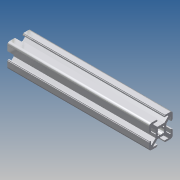
# Autodesk Inventor part: Motedius_20x20_B-Type_Slot-6_120
Saved by Autodesk Inventor 2015 SP1 (Build 190203100, 203)
## iProperties
Created: 2015-01-03
Part Number: Motedius_20x20_B-Type_Slot-6_120
Material: Aluminium 6061
Document SubType Name: Modeling
Designer: Marc
Mass: 190.994 g
Surface Area: 703.631 cm^2
Volume: 70.7386 cm^3
Density: 2.7 g/cm^3
Appearance: Aluminium - flach
Author: Marc
Autodesk Inventor part; units mm, degrees
ref_plane "YZ Plane" through (0, 0, 0) normal (1, 0, 0) x (0, 1, 0)
ref_plane "XZ Plane" through (0, 0, 0) normal (0, 1, 0) x (-1, 0, 0)
ref_plane "XY Plane" through (0, 0, 0) normal (0, 0, 1) x (1, 0, 0)
sketch "Skizze1" plane through (0, 0, 0) normal (1, 0, 0) x (0, 1, 0)
  line L0 (-14.5799, 0) -> (14.5799, 0) projected
  line L1 (0, -14.5799) -> (0, 14.5799) projected
  line L2 (9.5, 3) -> (9.5, 3.5)
  line L3 (9.5, 3.5) -> (10, 3.5)
  line L4 (8.5, 3) -> (8.5, 6.2861)
  line L5 (7.7861, 6.2861) -> (4.5, 3)
  line L6 (8.5, 6.2861) -> (7.7861, 6.2861)
  line L7 (8.5, 3) -> (9.5, 3)
  line L8 (9.5, -3) -> (9.5, -3.5)
  line L9 (9.5, -3.5) -> (10, -3.5)
  line L10 (8.5, -3) -> (8.5, -6.2861)
  line L11 (7.7861, -6.2861) -> (4.5, -3)
  line L12 (8.5, -6.2861) -> (7.7861, -6.2861)
  line L13 (8.5, -3) -> (9.5, -3)
  line L14 (10, 3.5) -> (10, 8)
  line L15 (10, -3.5) -> (10, -8)
  line L16 (-9.5, 3) -> (-9.5, 3.5)
  line L17 (-9.5, 3.5) -> (-10, 3.5)
  line L18 (-8.5, 3) -> (-8.5, 6.2861)
  line L19 (-7.7861, 6.2861) -> (-4.5, 3)
  line L20 (-8.5, 6.2861) -> (-7.7861, 6.2861)
  line L21 (-8.5, 3) -> (-9.5, 3)
  line L22 (-8.5, -3) -> (-9.5, -3)
  line L23 (-8.5, -3) -> (-8.5, -6.2861)
  line L24 (-8.5, -6.2861) -> (-7.7861, -6.2861)
  line L25 (-7.7861, -6.2861) -> (-4.5, -3)
  line L26 (-9.5, -3) -> (-9.5, -3.5)
  line L27 (-9.5, -3.5) -> (-10, -3.5)
  line L28 (3, -9.5) -> (3.5, -9.5)
  line L29 (3.5, -9.5) -> (3.5, -10)
  line L30 (3, -8.5) -> (6.2861, -8.5)
  line L31 (6.2861, -7.7861) -> (3, -4.5)
  line L32 (6.2861, -8.5) -> (6.2861, -7.7861)
  line L33 (3, -8.5) -> (3, -9.5)
  line L34 (-3, -8.5) -> (-3, -9.5)
  line L35 (-3, -8.5) -> (-6.2861, -8.5)
  line L36 (-6.2861, -8.5) -> (-6.2861, -7.7861)
  line L37 (-6.2861, -7.7861) -> (-3, -4.5)
  line L38 (-3, -9.5) -> (-3.5, -9.5)
  line L39 (-3.5, -9.5) -> (-3.5, -10)
  line L40 (3.5, 9.5) -> (3.5, 10)
  line L41 (3, 9.5) -> (3.5, 9.5)
  line L42 (3, 8.5) -> (3, 9.5)
  line L43 (3, 8.5) -> (6.2861, 8.5)
  line L44 (6.2861, 8.5) -> (6.2861, 7.7861)
  line L45 (6.2861, 7.7861) -> (3, 4.5)
  line L46 (-6.2861, 7.7861) -> (-3, 4.5)
  line L47 (-6.2861, 8.5) -> (-6.2861, 7.7861)
  line L48 (-3, 8.5) -> (-6.2861, 8.5)
  line L49 (-3, 8.5) -> (-3, 9.5)
  line L50 (-3, 9.5) -> (-3.5, 9.5)
  line L51 (-3.5, 9.5) -> (-3.5, 10)
  line L52 (8, 10) -> (3.5, 10)
  line L53 (-3.5, 10) -> (-8, 10)
  line L54 (-10, 8) -> (-10, 3.5)
  line L55 (-10, -3.5) -> (-10, -8)
  line L56 (-8, -10) -> (-3.5, -10)
  line L57 (3.5, -10) -> (8, -10)
  arc A0 (10, 8) -> (8, 10) centre (8, 8) ccw
  arc A1 (8, -10) -> (10, -8) centre (8, -8) ccw
  arc A2 (-10, -8) -> (-8, -10) centre (-8, -8) ccw
  arc A3 (-8, 10) -> (-10, 8) centre (-8, 8) ccw
  line L58 (-2.8201, 2.0744) -> (-2.113, 2.7815)
  line L59 (-2.113, 2.7815) -> (-1.5814, 2.2498)
  line L60 (-2.2813, 1.5356) -> (-2.8201, 2.0744)
  line L61 (2.8201, 2.0744) -> (2.113, 2.7815)
  line L62 (2.113, 2.7815) -> (1.5814, 2.2498)
  line L63 (2.2813, 1.5356) -> (2.8201, 2.0744)
  line L64 (2.0744, -2.8201) -> (2.7815, -2.113)
  line L65 (2.7815, -2.113) -> (2.2498, -1.5814)
  line L66 (1.5356, -2.2813) -> (2.0744, -2.8201)
  line L67 (-2.7815, -2.113) -> (-2.2498, -1.5814)
  line L68 (-2.0744, -2.8201) -> (-2.7815, -2.113)
  line L69 (-1.5356, -2.2813) -> (-2.0744, -2.8201)
  arc A4 (1.5814, 2.2498) -> (-1.5814, 2.2498) centre (0, 0) ccw
  arc A5 (1.5814, 2.2498) -> (-1.5814, 2.2498) centre (0, 0) ccw
  arc A6 (2.2498, -1.5814) -> (2.2813, 1.5356) centre (0, 0) ccw
  arc A7 (2.2498, -1.5814) -> (2.2813, 1.5356) centre (0, 0) ccw
  arc A8 (-2.2813, 1.5356) -> (-2.2498, -1.5814) centre (0, 0) ccw
  arc A9 (-1.5356, -2.2813) -> (1.5356, -2.2813) centre (0, 0) ccw
  arc A10 (-2.2813, 1.5356) -> (-2.2498, -1.5814) centre (0, 0) ccw
  arc A11 (-1.5356, -2.2813) -> (1.5356, -2.2813) centre (0, 0) ccw
  line L70 (0.3484, 4.5) -> (-0.0051, 4.1465)
  line L71 (-0.0051, 4.1465) -> (-0.3589, 4.5)
  line L72 (3, 4.5) -> (0.3484, 4.5)
  line L73 (-0.3589, 4.5) -> (-3, 4.5)
  line L74 (4.5, 0.3484) -> (4.1465, -0.0051)
  line L75 (4.1465, -0.0051) -> (4.5, -0.3589)
  line L76 (0.3484, -4.5) -> (-0.0051, -4.1465)
  line L77 (-0.0051, -4.1465) -> (-0.3589, -4.5)
  line L78 (-4.5, 0.3484) -> (-4.1465, -0.0051)
  line L79 (-4.1465, -0.0051) -> (-4.5, -0.3589)
  line L80 (4.5, 3) -> (4.5, 0.3484)
  line L81 (4.5, -0.3589) -> (4.5, -3)
  line L82 (3, -4.5) -> (0.3484, -4.5)
  line L83 (-0.3589, -4.5) -> (-3, -4.5)
  line L84 (-4.5, 3) -> (-4.5, 0.3484)
  line L85 (-4.5, -0.3589) -> (-4.5, -3)
  point P0 (-10, -10)
  point P1 (-10, 10)
  point P2 (10, -10)
  dimension "d0" = 20
  dimension "d1" = 20
  dimension "d4" = 6
  dimension "d9" = 0.5
  dimension "d10" = 0.5
  dimension "d13" = 45
  dimension "d14" = 3.2861
  dimension "d16" = 3
  dimension "d17" = 3.5
  dimension "d19" = 6
  dimension "d20" = 0.5
  dimension "d21" = 0.5
  dimension "d22" = 45
  dimension "d23" = 3.2861
  dimension "d25" = 2
  constraints: 168 end point, 35 parallel, 28 symmetric about line, 24 point on circle, 12 centre point, 10 perpendicular, 10 tangent, 8 point on line, 3 equal radius, 3 horizontal, 1 vertical
  measures "d0" distance of point (10, -10) point (-10, -10)
  measures "d1" distance of point (-10, -10) point (-10, 10)
  measures "d4" distance of L11.end L5.end
  measures "d9" distance of L2.end L3.end
  measures "d10" distance of L2.start L2.end
  measures "d13" angle of L5 L4
  measures "d14" distance of L4.start L4.end
  measures "d16" distance between parallel lines of L0 L7
  measures "d17" distance between parallel lines of L0 L3
  measures "d19" distance of L37.end L31.end
  measures "d20" distance of L29.end L28.end
  measures "d21" distance of L33.end L28.end
  measures "d22" angle of L31 L30
  measures "d23" distance of L30.start L32.start
  measures "d25" radius of A0
extrude "Extrusion1" add sketch "Skizze1" along normal mid plane 120 contours L78 L84 L19 L20 L18 L21 L16 L17 L54 A3 L53 L51 L50 L49 L48 L47 L46 L73 L71 L70 L1 A4 L59 L58 L60 A8 L0 | L0 A8 L67 L68 L69 A9 L1 L76 L77 L83 L37 L36 L35 L34 L38 L39 L56 A2 L55 L27 L26 L22 L23 L24 L25 L85 L79 L78 | A6 L63 L61 L62 A4 L1 L70 L72 L45 L44 L43 L42 L41 L40 L52 A0 L14 L3 L2 L7 L4 L6 L5 L80 L74 L0 | L0 L74 L75 L81 L11 L12 L10 L13 L8 L9 L15 A1 L57 L29 L28 L33 L30 L32 L31 L82 L76 L1 A9 L66 L64 L65 A6
